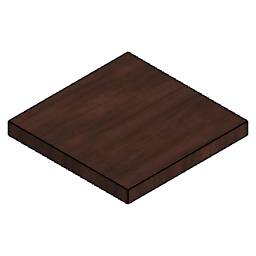
Table v2 (Autodesk Fusion 360 archive; units mm, degrees)
design "Table Top"
Autodesk Fusion 360 part; units mm, degrees
sketch "Sketch1" plane through (0, 0, 0) normal (0, 0, 1) x (1, 0, 0)
  line L0 (0, 50) -> (500, 50)
  line L1 (500, 50) -> (500, -450)
  line L2 (500, -450) -> (0, -450)
  line L3 (0, -450) -> (0, 50)
  dimension "d1" = 500
  dimension "d2" = 500
  constraint horizontal L0
  constraint vertical L1
  constraint horizontal L2
  constraint vertical L3
  measures "d1" distance of L0.start L0.end
  measures "d2" distance of L0.start L2.end
extrude "Extrude1" add sketch "Sketch1" along normal blind 50
sketch "Sketch2" plane through (0, 0, 0) normal (0, 0, -1) x (1, 0, 0)
  line L0 (500, 450) -> (0, 450)
  line L1 (0, 450) -> (0, -50)
  line L2 (0, -50) -> (500, -50)
  line L3 (500, -50) -> (500, 450)
  circle A0 centre (475, 425) radius 10
  dimension "d5" = 20
  dimension "d6" = 25
  dimension "d7" = 25
  measures "d5" diameter of A0
  measures "d6" distance of L0 A0.centre
  measures "d7" distance of L3 A0.centre
extrude "Extrude2" cut sketch "Sketch2" against normal blind 20 contours A0
sketch "Sketch3" plane through (0, 0, 0) normal (0, 0, -1) x (1, 0, 0)
  circle A0 centre (475, 425) radius 10
  line L0 (500, 450) -> (0, 450)
  line L1 (0, 450) -> (0, -50)
  line L2 (0, -50) -> (500, -50)
  line L3 (500, -50) -> (500, 450)
  circle A1 centre (25, 425) radius 10
  dimension "d10" = 20
  dimension "d11" = 25
  dimension "d12" = 25
  measures "d10" diameter of A1
  measures "d11" distance of L0 A1.centre
  measures "d12" distance of L1 A1.centre
extrude "Extrude3" cut sketch "Sketch3" against normal blind 20 contours A1
sketch "Sketch4" plane through (0, 0, 0) normal (0, 0, -1) x (1, 0, 0)
  circle A0 centre (25, 425) radius 10
  circle A1 centre (475, 425) radius 10
  line L0 (500, 450) -> (0, 450)
  line L1 (0, 450) -> (0, -50)
  line L2 (0, -50) -> (500, -50)
  line L3 (500, -50) -> (500, 450)
  circle A2 centre (25, -25) radius 10
  dimension "d15" = 20
  dimension "d16" = 500
  dimension "d17" = 25
  dimension "d18" = 25
  measures "d15" diameter of A2
  measures "d16" distance of L0.end L1.end
  measures "d17" distance of L1 A2.centre
  measures "d18" distance of L2 A2.centre
extrude "Extrude4" cut sketch "Sketch4" against normal blind 20 contours A2
sketch "Sketch5" plane through (0, 0, 0) normal (0, 0, -1) x (1, 0, 0)
  circle A0 centre (25, -25) radius 10
  circle A1 centre (25, 425) radius 10
  circle A2 centre (475, 425) radius 10
  line L0 (500, 450) -> (0, 450)
  line L1 (0, 450) -> (0, -50)
  line L2 (0, -50) -> (500, -50)
  line L3 (500, -50) -> (500, 450)
  circle A3 centre (475, -25) radius 10
  dimension "d21" = 20
  dimension "d22" = 25
  dimension "d23" = 25
  measures "d21" diameter of A3
  measures "d22" distance of L3 A3.centre
  measures "d23" distance of L2 A3.centre
extrude "Extrude5" cut sketch "Sketch5" against normal blind 20 contours A3

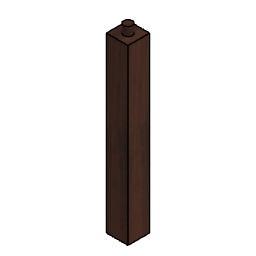
design "Leg"
Autodesk Fusion 360 part; units mm, degrees
sketch "Sketch1" plane through (0, 0, 0) normal (0, 0, 1) x (1, 0, 0)
  line L0 (0, 50) -> (50, 50)
  line L1 (50, 50) -> (50, 0)
  line L2 (50, 0) -> (0, 0)
  line L3 (0, 0) -> (0, 50)
  dimension "d1" = 50
  dimension "d2" = 50
  constraint horizontal L0
  constraint vertical L1
  constraint horizontal L2
  constraint vertical L3
  measures "d1" distance of L0.start L0.end
  measures "d2" distance of L0.start L2.end
extrude "Extrude1" add sketch "Sketch1" along normal blind 400
sketch "Sketch2" plane through (0, 0, 400) normal (0, 0, 1) x (-1, 0, 0)
  line L0 (0, 0) -> (-50, 0)
  line L1 (-50, 0) -> (-50, -50)
  line L2 (-50, -50) -> (0, -50)
  line L3 (0, -50) -> (0, 0)
  circle A0 centre (-25, -25) radius 10
  dimension "d5" = 20
  dimension "d6" = 25
  dimension "d7" = 25
  measures "d5" diameter of A0
  measures "d6" distance of L2 A0.centre
  measures "d7" distance of L3 A0.centre
extrude "Extrude2" add sketch "Sketch2" along normal blind 20 contours A0
